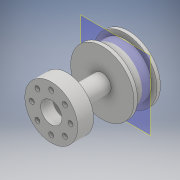
# Autodesk Inventor part: spinning_wheel
Saved by Autodesk Inventor 2018 (Build 220112000, 112)
## iProperties
Created: 2019-05-24
Part Number: spinning_wheel
Material: Generic
Document SubType Name: Modeling
Designer: bitbots
Density: 1 g/cm^3
Appearance: Default
Author: bitbots
Autodesk Inventor part; units mm, degrees
ref_plane "YZ Plane" through (0, 0, 0) normal (1, 0, 0) x (0, 1, 0)
ref_plane "XZ Plane" through (0, 0, 0) normal (0, 1, 0) x (-1, 0, 0)
ref_plane "XY Plane" through (0, 0, 0) normal (0, 0, 1) x (1, 0, 0)
sketch "Sketch1" plane through (0, 0, 0) normal (0, 1, 0) x (-1, 0, 0)
  circle A0 centre (0, 0) radius 15
  dimension "d0" = 30
  constraints: 1 centre point, 1 coincident
  measures "d0" diameter of A0
extrude "Extrusion1" add sketch "Sketch1" along normal blind 9
sketch "Sketch3" plane through (0, 9, 0) normal (0, 1, 0) x (1, 0, 0)
  circle A0 centre (0, 0) radius 11 construction
  line L0 (0, 0) -> (0, 11) construction
  line L1 (0, 11) -> (7.7782, 7.7782) construction
  line L2 (7.7782, 7.7782) -> (11, 0) construction
  line L3 (11, 0) -> (7.7782, -7.7782) construction
  line L4 (7.7782, -7.7782) -> (0, -11) construction
  line L5 (0, -11) -> (-7.7782, -7.7782) construction
  line L6 (-7.7782, -7.7782) -> (-11, 0) construction
  line L7 (-11, 0) -> (-7.7782, 7.7782) construction
  line L8 (-7.7782, 7.7782) -> (0, 11) construction
  circle A1 centre (-11, 0) radius 1.4
  circle A2 centre (-7.7782, 7.7782) radius 1.4
  circle A3 centre (-7.7782, -7.7782) radius 1.4
  circle A4 centre (0, -11) radius 1.4
  circle A5 centre (7.7782, -7.7782) radius 1.4
  circle A6 centre (11, 0) radius 1.4
  circle A7 centre (7.7782, 7.7782) radius 1.4
  circle A8 centre (0, 11) radius 1.4
  dimension "d12" = 22
  dimension "d13" = 2.8
  dimension "d14" = 2.8
  dimension "d15" = 2.8
  dimension "d16" = 2.8
  dimension "d17" = 2.8
  dimension "d18" = 2.8
  dimension "d19" = 2.8
  dimension "d20" = 2.8
  constraints: 18 end point, 10 coincident, 8 centre point, 1 vertical, 1 vertical alignment, 19 other
  measures "d13" diameter of A1
  measures "d14" diameter of A2
  measures "d15" diameter of A3
  measures "d16" diameter of A4
  measures "d17" diameter of A5
  measures "d18" diameter of A6
  measures "d19" diameter of A7
  measures "d20" diameter of A8
extrude "Extrusion3" cut sketch "Sketch3" against normal up to next
sketch "Sketch4" plane through (0, 9, 0) normal (0, 1, 0) x (1, 0, 0)
  circle A0 centre (-11, 0) radius 1.4 construction
  circle A1 centre (0, 0) radius 11 construction
  line L0 (0, 0) -> (-11, 0) construction
  line L1 (-11, 0) -> (-7.7782, 7.7782) construction
  line L2 (-7.7782, 7.7782) -> (0, 11) construction
  line L3 (0, 11) -> (7.7782, 7.7782) construction
  line L4 (7.7782, 7.7782) -> (11, 0) construction
  line L5 (11, 0) -> (7.7782, -7.7782) construction
  line L6 (7.7782, -7.7782) -> (0, -11) construction
  line L7 (0, -11) -> (-7.7782, -7.7782) construction
  line L8 (-7.7782, -7.7782) -> (-11, 0) construction
  circle A2 centre (-11, 0) radius 2.6
  circle A3 centre (-7.7782, 7.7782) radius 1.4 projected
  circle A4 centre (-7.7782, 7.7782) radius 2.6
  circle A5 centre (0, 11) radius 2.6
  circle A6 centre (7.7782, 7.7782) radius 2.6
  circle A7 centre (11, 0) radius 2.6
  circle A8 centre (7.7782, -7.7782) radius 1.4 projected
  circle A9 centre (7.7782, -7.7782) radius 2.6
  circle A10 centre (0, -11) radius 1.4 projected
  circle A11 centre (0, -11) radius 2.6
  circle A12 centre (-7.7782, -7.7782) radius 2.6
  dimension "d23" = 5.2
  dimension "d24" = 5.2
  dimension "d25" = 5.2
  dimension "d26" = 5.2
  dimension "d27" = 5.2
  dimension "d28" = 5.2
  dimension "d29" = 5.2
  dimension "d30" = 5.2
  constraints: 18 end point, 10 coincident, 8 centre point, 1 horizontal, 1 horizontal alignment, 19 other
  measures "d23" diameter of A2
  measures "d24" diameter of A4
  measures "d25" diameter of A5
  measures "d26" diameter of A6
  measures "d27" diameter of A7
  measures "d28" diameter of A9
  measures "d29" diameter of A11
  measures "d30" diameter of A12
extrude "Extrusion4" cut sketch "Sketch4" against normal blind 3.5
sketch "Sketch5" plane through (0, 0, 0) normal (0, -1, 0) x (1, 0, 0)
  circle A0 centre (0, 0) radius 6
  dimension "d33" = 12
  constraints: 1 centre point, 1 coincident
  measures "d33" diameter of A0
extrude "Extrusion5" cut sketch "Sketch5" against normal blind 7
sketch "Skizze6" plane through (0, 9, 0) normal (0, 1, 0) x (1, 0, 0)
  circle A0 centre (0, 0) radius 6 projected
  circle A1 centre (0, 0) radius 5
  dimension "d36" = 10
  constraints: 1 centre point, 1 coincident
  measures "d36" diameter of A1
extrude "Extrusion6" add sketch "Skizze6" along normal blind 20 contours A1
sketch "Skizze9" plane through (0, 29, 0) normal (0, 1, 0) x (1, 0, 0)
  circle A0 centre (0, 0) radius 15 construction
  circle A1 centre (0, 0) radius 6 construction
  line L0 (0, 0) -> (0, -15) construction
  line L1 (0, 0) -> (0, -15) construction
  circle A2 centre (0, 0) radius 15
  constraints: 4 end point, 2 vertical, 2 vertical alignment, 1 coincident, 3 other
extrude "Extrusion7" add sketch "Skizze9" along normal blind 15
sketch "Skizze10" plane through (0, 44, 0) normal (0, 1, 0) x (1, 0, 0)
  line L0 (0, 0) -> (0, -18) construction
  circle A0 centre (0, 0) radius 5 projected
  circle A1 centre (0, 0) radius 18
  dimension "d44" = 18
  constraints: 2 end point, 1 coincident, 1 vertical, 1 vertical alignment, 2 other
  measures "d44" distance of L0.start L0.end
extrude "Extrusion8" add sketch "Skizze10" against normal blind 2
ref_plane "Arbeitsebene2" through (0, 36.5, 0) normal (0, 1, 0) x (1, 0, 0)
mirror "Spiegeln1" about plane through (0, 36.5, 0) normal (0, 1, 0) of "Extrusion8"
body "Solid1"
